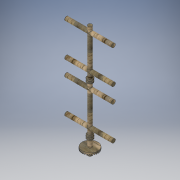
# Autodesk Inventor part: Sailbeam
Saved by Autodesk Inventor 2018.1 (Build 221171000, 171)
## iProperties
Created: 2017-09-02
Part Number: Sailbeam
Material: Generic
Document SubType Name: Modeling
Designer: ToreDenStore
Density: 1 g/cm^3
Appearance: Default
Author: ToreDenStore
Autodesk Inventor part; units mm, degrees
ref_plane "YZ Plane" through (0, 0, 0) normal (1, 0, 0) x (0, 1, 0)
ref_plane "XZ Plane" through (0, 0, 0) normal (0, 1, 0) x (-1, 0, 0)
ref_plane "XY Plane" through (0, 0, 0) normal (0, 0, 1) x (1, 0, 0)
sketch "Sketch1" plane through (0, 0, 0) normal (0, 1, 0) x (-1, 0, 0)
  circle A0 centre (0, 0) radius 5
  dimension "d0" = 10
  constraints: 1 centre point, 1 coincident
  measures "d0" diameter of A0
extrude "Extrusion1" add sketch "Sketch1" along normal blind 287
ref_plane "Work Plane1" through (0, 40, 0) normal (0, -1, 0) x (1, 0, 0)
sketch "Sketch2" plane through (0, 40, 0) normal (0, -1, 0) x (1, 0, 0)
  circle A0 centre (0, 0) radius 7.5
  circle A1 centre (0, 0) radius 5 projected
  dimension "d4" = 15
  constraints: 1 centre point, 1 coincident
  measures "d4" diameter of A0
extrude "Extrusion2" add sketch "Sketch2" along normal blind 3
ref_plane "Work Plane2" through (0, 41.5, 0) normal (0, 1, 0) x (1, 0, 0)
mirror "Mirror1" about plane through (0, 41.5, 0) normal (0, 1, 0) of "Extrusion2"
ref_plane "Work Plane3" through (0, 104, 0) normal (0, -1, 0) x (1, 0, 0)
mirror "Mirror2" about plane through (0, 104, 0) normal (0, -1, 0) of "Extrusion2", "Mirror1"
ref_plane "Work Plane4" through (0, 18.5, 0) normal (0, 1, 0) x (1, 0, 0)
sketch "Sketch3" plane through (0, 18.5, 0) normal (0, 1, 0) x (1, 0, 0)
  circle A0 centre (0, 0) radius 5 projected
  circle A1 centre (0, 0) radius 20
  dimension "d10" = 40
  constraints: 1 centre point, 1 coincident
  measures "d10" diameter of A1
extrude "Extrusion3" add sketch "Sketch3" against normal blind 3
sketch "Sketch4" plane through (0, 15.5, 0) normal (0, 1, 0) x (1, 0, 0)
  circle A0 centre (0, 0) radius 20 projected
  line L0 (0, 0) -> (-1.5285, 16.9311) construction
  line L1 (0, 20) -> (0, 17)
  arc A1 (-1.5285, 16.9311) -> (0, 17) centre (0, 0) ccw construction
  line L2 (-1.5285, 16.9311) -> (-1.7982, 19.919)
  line L3 (0, 17) -> (0, 0) construction
  arc A2 (0, 17) -> (-1.5285, 16.9311) centre (0, 0) ccw
  line L4 (0, 28) -> (0, -28) construction
  dimension "d13" = 1.8
  dimension "d14" = 3
  dimension "d15" = 0
  constraints: 8 end point, 6 point on circle, 2 centre point, 2 collinear, 1 coincident
  measures "d13" distance of L2.end L1.start
  measures "d14" radial gap between concentric circles of A0 A1
  measures "d15" distance between parallel lines of L1 L4
extrude "Extrusion4" add sketch "Sketch4" against normal blind 3 contours L1 A2 L2 A0 picked at (-1.3392, 18.9508)
chamfer "Chamfer1" distance 1 angle 30 1 edges at (0, 12.5, -18.5) measured on face at (0, 13, -18.5)
chamfer "Chamfer2" distance 1 angle 30 1 edges at (-1.6633, 12.5, -18.4251) measured on face at (-1.6633, 13, -18.4251)
fillet "Fillet2" radius 3 2 edges at (0, 13.5, -18.5) (-1.6633, 13.5, -18.4251)
pattern_circular "Circular Pattern1" count 32 over 360 about axis through (0, 0, 0) along (0, 1, 0) of "Extrusion4", "Chamfer1", "Chamfer2", "Fillet2"
ref_plane "Work Plane5" through (0, 61, 0) normal (0, 1, 0) x (1, 0, 0)
sketch "Sketch5" plane through (0, 61, 0) normal (0, 1, 0) x (1, 0, 0)
  line L0 (-60, 0) -> (60, 0)
  line L1 (60, 0) -> (60, -5)
  line L2 (60, -5) -> (-60, -5)
  line L3 (-60, -5) -> (-60, 0)
  point P0 (0, 0)
  dimension "d28" = 5
  dimension "d29" = 120
  dimension "d30" = 60
  dimension "d31" = 0
  constraints: 8 end point, 2 parallel, 1 horizontal, 1 perpendicular
  measures "d28" distance of L0.end L1.end
  measures "d29" distance of L0.start L0.end
  measures "d30" distance from line of point (0, 0) L1
  measures "d31" distance from line of point (0, 0) L0
revolve "Revolution1" add sketch "Sketch5" angle 360 about axis through (-60, 61, 0) along (1, 0, 0)
ref_plane "Work Plane6" through (0, 104, 0) normal (0, 1, 0) x (1, 0, 0)
mirror "Mirror3" about plane through (0, 104, 0) normal (0, 1, 0) of "Revolution1"
ref_plane "Work Plane7" through (0, 166.5, 0) normal (0, 1, 0) x (1, 0, 0)
mirror "Mirror4" about plane through (0, 166.5, 0) normal (0, 1, 0) of "Revolution1", "Mirror3"
equation "\"d30\" = 0.5 * d29"
body "Solid1"
